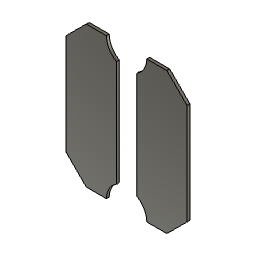
Template v1 (Autodesk Fusion 360 design; units mm, degrees)
Autodesk Fusion 360 part; units mm, degrees
sketch "Sketch1" plane through (0, 0, 0) normal (0, 1, 0) x (1, 0, 0)
  line L0 (-50, 0) -> (-100, 0)
  line L1 (-150, -300) -> (-100, -350)
  arc A0 (50, -350) -> (0, -300) centre (0, -350) ccw
  arc A1 (0, -300) -> (-50, -350) centre (0, -350) ccw
  line L2 (100, 0) -> (150, -50)
  line L3 (-100, -350) -> (-50, -350)
  line L4 (-150, -50) -> (-150, -300)
  line L5 (150, -50) -> (150, -300)
  line L6 (-100, 0) -> (-150, -50)
  line L7 (100, -350) -> (50, -350)
  line L8 (50, 0) -> (100, 0)
  line L9 (150, -300) -> (100, -350)
  arc A2 (-50, 0) -> (0, -50) centre (0, 0) ccw
  arc A3 (0, -50) -> (50, 0) centre (0, 0) ccw
  point P0 (0, -175)
  dimension "d1" = 100
  dimension "d2" = 50
  dimension "d3" = 250
  dimension "d4" = 100
  constraint coincident A2.centre A3.centre
  constraint horizontal L0
  constraint vertical L4
  constraint horizontal L3
  measures "d1" diameter of A2
  measures "d2" distance of L0.end L0.start
  measures "d3" distance of L4.start L1.start
  measures "d4" diameter of A1
extrude "Extrude1" add sketch "Sketch1" along normal blind 7 makes body 1
sketch "Sketch2" plane through (0, 0, 0) normal (0, -1, 0) x (1, 0, 0)
  line L0 (-100, 0) -> (-50, 0)
  arc A0 (50, 0) -> (-50, 0) centre (0, 0) ccw
  line L1 (50, 0) -> (100, 0)
  line L2 (100, 0) -> (150, 50)
  line L3 (150, 50) -> (150, 300)
  line L4 (150, 300) -> (100, 350)
  line L5 (100, 350) -> (50, 350)
  arc A1 (-50, 350) -> (50, 350) centre (0, 350) ccw
  line L6 (-50, 350) -> (-100, 350)
  line L7 (-100, 350) -> (-150, 300)
  line L8 (-150, 300) -> (-150, 50)
  line L9 (-150, 50) -> (-100, 0)
  line L10 (-25, 350) -> (25, 350)
  line L11 (25, 350) -> (25, 0)
  line L12 (25, 0) -> (-25, 0)
  line L13 (-25, 0) -> (-25, 350)
  line L14 (-25, 350) -> (25, 0) construction
  line L15 (25, 350) -> (-25, 0) construction
  point P0 (0, 175)
  point P1 (0, 175)
  dimension "d10" = 50
  dimension "d11" = 350
  constraint horizontal L10
  constraint perpendicular L10 L11
  constraint parallel L10 L12
  constraint parallel L11 L13
  constraint coincident L14 P1
  constraint coincident L15 P1
  constraint coincident P1 P0
  measures "d10" distance of L11.end L12.end
  measures "d11" distance of L10.end L11.end
extrude "Extrude2" cut sketch "Sketch2" against normal blind 7 contours A0 A1 L11 L13 | A0 L11 L12 L13 | A1 L10 L11 L13 bodies 1 makes body 2 at (66.6667, 0, 216.6667)
sketch "Sketch3" plane through (0, 0, 350) normal (0, 0, 1) x (-1, 0, 0)
  line L0 (-50, 0) -> (-100, 0)
  line L1 (-100, 0) -> (-100, -7)
  line L2 (-100, -7) -> (-50, -7)
  line L3 (-50, -7) -> (-50, 0)
  line L4 (-50, -3.5) -> (50, -3.5)
  point P0 (0, -3.5)
  constraint midpoint L3 L4.start
  constraint perpendicular L3 L4
  constraint midpoint L4 P0
sketch "Sketch4" plane through (0, 0, 0) normal (1, 0, 0) x (0, 1, 0)
  line L0 (3.5, 350) -> (-50.9682, 342.3702) construction
  line L1 (3.5, 350) -> (58.5, 350) construction
  point P0 (3.5, 350)
  dimension "d15" = 172.026
  dimension "d16" = 55
  constraint horizontal L1
  constraint coincident P0 L0.start
  measures "d15" angle of L0 L1
  measures "d16" distance of P0 L0.end
ref_plane "WorkPlane1" through (0, -23.7341, 346.1851) normal (0, -0.138724, 0.990331) x (0, -0.990331, -0.138724)
sketch "Sketch5" plane through (0, 0, 0) normal (0, 1, 0) x (1, 0, 0)
chamfer "Chamfer1" [suppressed]
equation "d15 = 180 deg - 7.974 deg"
